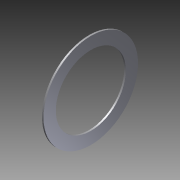
# Autodesk Inventor part: WML5010ZZ Shield
Saved by Autodesk Inventor 2013 SP2 (Build 170200200, 200)
## iProperties
Category: PARTsolutions
Company: KOYO
Created: 2013-06-21
Part Number: WML5010ZZ Shield
Catalog Web Link: www.cadenas.de
Description: Open ball s-
Vendor: KOYO
Document SubType Name: Modeling
Designer: PARTuser1
Manufacturer: KOYO
Density: 1 g/cm^3
Material: Generic
PSOL_IDENT_0: {$CADENAS_DATA\23d-libs\koyo\deep_groove_ball_bearings\extra_small_bb_miniature_bb\extra_small_bb_mi
PSOL_IDENT_1: niature_bb\open_shield.prj},181 {VTYP=3D},{NB=WML5010ZZ Shield},{LINA=WML5010ZZ Shield},{NN=Open bal
PSOL_IDENT_2: l s},{DATE=26.11.2007 07:28:04},{GEOMDATE=26.11.2007 00:00:00},{VERSION=},{LINEID=1000},{LINESUBID=-
PSOL_IDENT_3: 1},{WBVAR=}  {NB=WML5010ZZ Shield},{LINA=WML5010ZZ Shield},{KT=DUMMY},{SRS=BS},{TP=60},{SD=5.0},{D=1
PSOL_IDENT_4: 0},{B=4.0},{R=0.10},{ST=2-D},{ORDER=WML5010ZZ},{VERS1=2.0},{NAME=Shield},{C=0.43},{C0=0.17},{NG=5500
PSOL_IDENT_5: 0},{NO=0},{SR=0.20},{DF1=0.0},{BF1=0.0},{BD=1.20},{PCD=7.35},{ID=6.45},{OD=8.25},{GID=6.45},{GOD=8.7
PSOL_IDENT_6: 0},{X1=0.36},{X2=0.15},{NOB=10}
CNS_NB: WML5010ZZ Shield
CNS_NBSYN: $ORDER. $NAME.
CNS_LINA: WML5010ZZ Shield
CNS_SRS: BS
CNS_TP: 60
CNS_SD: 5.0
CNS_D: 10
CNS_B: 4.0
CNS_R: 0.10
CNS_ST: 2-D
CNS_ORDER: WML5010ZZ
CNS_VERS1: 2.0
CNS_NAME: Shield
CNS_C: 0.43
CNS_C0: 0.17
CNS_NG: 55000
CNS_NO: 0
CNS_SR: 0.20
CNS_DF1: 0.0
CNS_BF1: 0.0
CNS_BD: 1.20
CNS_PCD: 7.35
CNS_ID: 6.45
CNS_OD: 8.25
CNS_GID: 6.45
CNS_GOD: 8.70
CNS_X1: 0.36
CNS_X2: 0.15
CNS_NOB: 10
SUPPLIER: KOYO
ARTICLENO: WML5010ZZ Shield
BOMINFO: WML5010ZZ Shield
CREATOR: CADENAS GmbH
Title: WML5010ZZ Shield
Author: Cadenas PARTsolutions
Autodesk Inventor part; units mm, degrees
sketch "Sketch_1" plane through (0, 0, 0) normal (0, 0, 1) x (1, 0, 0)
  line L0 (0.36, 0) -> (0.21, 0)
  line L1 (0.21, 3.225) -> (0.36, 3.225)
  line L2 (0.36, 3.225) -> (0.36, 4.35)
  line L3 (0.36, 4.35) -> (0.21, 4.35)
  line L4 (0.21, 4.35) -> (0.21, 3.225)
  constraints: 10 end point
revolve "Revolution1" add sketch "Sketch_1" angle 360 about axis through (0.36, 0, 0) along (1, 0, 0)
ref_plane "ring_XY" through (0, 0, 0) normal (1, 0, 0) x (0, 0, -1)
ref_plane "ring_YZ" through (0, 0, 0) normal (0, 0, -1) x (0, 1, 0)
ref_plane "ring_ZX" through (0, 0, 0) normal (0, 1, 0) x (1, 0, 0)
body "Solid1"
